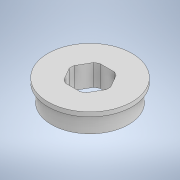
# Autodesk Inventor part: part_ Ball Bearing for Thundershaft
Saved by Autodesk Inventor 2021.1 (Build 251245000, 245)
## iProperties
Created: 2020-01-15
Part Number: part_ Ball Bearing for Thundershaft
Material: Generic
Document SubType Name: Modeling
Designer: aidan
Density: 1 g/cm^3
Appearance: Default
Author: aidan
Autodesk Inventor part; units mm, degrees
ref_plane "YZ Plane" through (0, 0, 0) normal (1, 0, 0) x (0, 1, 0)
ref_plane "XZ Plane" through (0, 0, 0) normal (0, 1, 0) x (-1, 0, 0)
ref_plane "XY Plane" through (0, 0, 0) normal (0, 0, 1) x (1, 0, 0)
sketch "Sketch5" plane through (0, 0, 0) normal (0, 0, 1) x (1, 0, 0)
  line L0 (0, 0) -> (0, 6.35)
  line L1 (0, 6.35) -> (-1.27, 6.35)
  line L2 (-1.27, 6.35) -> (-1.27, 7.9502)
  line L3 (-1.27, 7.9502) -> (29.845, 7.9502)
  line L4 (29.845, 7.9502) -> (29.845, 6.35)
  line L5 (29.845, 6.35) -> (28.575, 6.35)
  line L6 (28.575, 6.35) -> (28.575, 0)
  line L7 (28.575, 0) -> (0, 0)
  line L8 (14.2875, 0) -> (14.2875, 7.9502)
  dimension "d8" = 28.575
  dimension "d9" = 31.115
  dimension "d10" = 6.35
  dimension "d12" = 7.9502
  constraints: 18 end point, 6 perpendicular, 2 midpoint, 2 point on line, 1 collinear, 1 vertical
  measures "d8" distance between parallel lines of L6 L0
  measures "d9" distance between parallel lines of L4 L2
  measures "d10" distance of L5.end L6.end
  measures "d12" distance between parallel lines of L7 L3
revolve "Revolution2" add sketch "Sketch5" angle 360 about axis through (14.2875, 0, 0) along (0, 1, 0) contours L0 L1 L2 L3 L8 L7
sketch "Sketch6" plane through (14.2875, 7.9502, 0) normal (0, 1, 0) x (1, 0, 0)
  line L0 (-7.3323, 0) -> (-3.6662, 6.35)
  line L1 (-3.6662, 6.35) -> (3.6662, 6.35)
  line L2 (3.6662, 6.35) -> (7.3323, 0)
  line L3 (7.3323, 0) -> (3.6662, -6.35)
  line L4 (3.6662, -6.35) -> (-3.6662, -6.35)
  line L5 (-3.6662, -6.35) -> (-7.3323, 0)
  circle A0 centre (0, 0) radius 15.5575 projected
  circle A1 centre (0, 0) radius 6.8758
  point P0 (-14.2875, 0)
  point P1 (2.637, -6.35)
  point P2 (4.1808, -5.4587)
  point P3 (6.8178, -0.8913)
  point P4 (6.8178, 0.8913)
  point P5 (4.1808, 5.4587)
  point P6 (2.637, 6.35)
  point P7 (-2.637, 6.35)
  point P8 (-4.1808, 5.4587)
  point P9 (-6.8178, 0.8913)
  point P10 (-6.8178, -0.8913)
  point P11 (-4.1808, -5.4587)
  point P12 (-2.637, -6.35)
  dimension "d14" = 12.7
  dimension "d15" = 13.7516
  constraints: 12 end point, 2 coincident, 1 centre point, 1 horizontal, 13 other
  measures "d14" distance between parallel lines of L4 L1
  measures "d15" diameter of A1
extrude "Extrusion1" cut sketch "Sketch6" against normal through all contours L0 A1 L1 L2 L3 L4 L5
body "Solid2"
